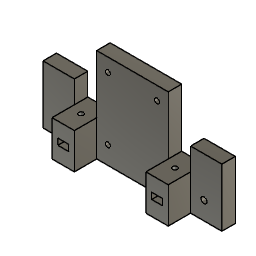
Y axis wheel frame v1 (Autodesk Fusion 360 design; units mm, degrees)
Autodesk Fusion 360 part; units mm, degrees
note: some values were not read from the file. Set by a fixed rule: which face or edge a step refers to.
sketch "Sketch1" plane through (0, 0, 0) normal (0, 1, 0) x (1, 0, 0)
  circle A0 centre (80, -25) radius 3.3
  circle A1 centre (-80, -25) radius 3.3
  line L0 (-100, -45) -> (-100, -5)
  line L1 (-100, -5) -> (100, -5)
  line L2 (100, -5) -> (100, -45)
  circle A2 centre (-80, -25) radius 6.55 construction
  circle A3 centre (80, -25) radius 6.55 construction
  line L3 (-65, -45) -> (-40, -45)
  line L4 (-40, -45) -> (-40, -5)
  line L5 (-40, -5) -> (-65, -5)
  line L6 (-65, -5) -> (-65, -45)
  line L7 (65, -45) -> (40, -45)
  line L8 (40, -45) -> (40, -5)
  line L9 (40, -5) -> (65, -5)
  line L10 (65, -5) -> (65, -45)
  line L11 (-40, -25) -> (-27.5, -25) construction
  line L12 (40, -25) -> (27.5, -25) construction
  circle A4 centre (-27.5, -25) radius 2.75
  circle A5 centre (27.5, -25) radius 2.75
  line L13 (-27.5, -25) -> (-27.5, -95) construction
  line L14 (27.5, -25) -> (27.5, -95) construction
  circle A6 centre (27.5, -95) radius 2.75
  circle A7 centre (-27.5, -95) radius 2.75
  line L15 (40, -45) -> (40, -105)
  line L16 (40, -105) -> (-40, -105)
  line L17 (-40, -105) -> (-40, -45)
  line L18 (-100, -45) -> (-65, -45)
  line L19 (65, -45) -> (100, -45)
  dimension "d3" = 160
  dimension "d4" = 6.6
  dimension "d5" = 6.6
  dimension "d6" = 13.1
  dimension "d7" = 13.1
  dimension "d11" = 12.5
  dimension "d12" = 12.5
  dimension "d13" = 5.5
  dimension "d14" = 5.5
  dimension "d15" = 70
  dimension "d16" = 70
  dimension "d17" = 5.5
  dimension "d18" = 5.5
  constraint vertical L0
  constraint horizontal L1
  constraint vertical L2
  constraint concentric A1 A2
  constraint concentric A0 A3
  constraint horizontal L3
  constraint vertical L4
  constraint horizontal L5
  constraint vertical L6
  constraint coincident L1 L4.end
  constraint horizontal L7
  constraint vertical L8
  constraint horizontal L9
  constraint vertical L10
  constraint coincident L1 L8.end
  constraint midpoint L4 L11.start
  constraint perpendicular L4 L11
  constraint midpoint L8 L12.start
  constraint perpendicular L8 L12
  constraint coincident L11.end A4.centre
  constraint coincident L12.end A5.centre
  constraint perpendicular L11 L13
  constraint coincident L14.end A6.centre
  constraint coincident L13.end A7.centre
  constraint vertical L15
  constraint horizontal L16
  constraint vertical L17
  constraint perpendicular L6 L18
  constraint perpendicular L2 L19
  measures "d3" distance of A0.centre A1.centre
  measures "d4" diameter of A0
  measures "d5" diameter of A1
  measures "d6" diameter of A2
  measures "d7" diameter of A3
  measures "d11" distance of L11.start L11.end
  measures "d12" distance of L12.start L12.end
  measures "d13" diameter of A4
  measures "d14" diameter of A5
  measures "d15" distance of L11.end L13.end
  measures "d16" distance of L12.end L14.end
  measures "d17" diameter of A6
  measures "d18" diameter of A7
extrude "Extrude1" add sketch "Sketch1" along normal blind 15
extrude "Extrude2" add sketch "Sketch1" against normal blind 85 contours L1 L3 L4 L5 L6 | L1 L7 L8 L9 L10
sketch "Sketch2" plane through (0, 0, 45) normal (0, 0, 1) x (-1, 0, 0)
  line L0 (100, 0) -> (65, 0)
  line L1 (65, 0) -> (65, 85)
  line L2 (65, 85) -> (40, 85)
  line L3 (40, 85) -> (40, 0)
  line L4 (40, 0) -> (40, -15)
  line L5 (40, -15) -> (100, -15)
  line L6 (100, -15) -> (100, 0)
  line L7 (65, 0) -> (40, 0) construction
  line L8 (52.5, -15) -> (52.5, 5) construction
  line L9 (52.5, 5) -> (52.5, 75) construction
  dimension "d23" = 20
  dimension "d24" = 70
  constraint coincident L0.end L1.start
  constraint coincident L3.end L4.start
  constraint coincident L5 L8.start
  constraint perpendicular L7 L8
  constraint parallel L8 L9
  measures "d23" distance of L8.start L8.end
  measures "d24" distance of L8.end L9.end
sketch "Sketch3" plane through (0, 0, 45) normal (0, 0, 1) x (-1, 0, 0)
  line L0 (-65, 0) -> (-100, 0)
  line L1 (-100, 0) -> (-100, -15)
  line L2 (-100, -15) -> (-40, -15)
  line L3 (-40, -15) -> (-40, 0)
  line L4 (-40, 0) -> (-40, 85)
  line L5 (-40, 85) -> (-65, 85)
  line L6 (-65, 85) -> (-65, 0)
  line L7 (-65, 0) -> (-40, 0) construction
  line L8 (-52.5, -15) -> (-52.5, 5) construction
  line L9 (-52.5, 5) -> (-52.5, 75) construction
  dimension "d25" = 20
  dimension "d26" = 70
  constraint coincident L0.start L6.end
  constraint coincident L3.end L4.start
  constraint coincident L2 L8.start
  constraint perpendicular L2 L8
  constraint perpendicular L2 L9
  measures "d25" distance of L8.start L8.end
  measures "d26" distance of L8.end L9.end
hole "Hole1" at (-52.5, -5, 45) at (52.5, -5, 45) direction (0, 0, -1) diameter 5.5 depth 40 tip angle 180
extrude "Extrude3" cut 2 faces at (-56.6667, -85, 18.3333) (48.3333, -85, 18.3333) along direction (0, 1, 0) blind 65
extrude "Extrude4" add 2 faces at (-56.6667, -20, 18.3333) (48.3333, -20, 18.3333) along direction (0, -1, 0) blind 5
extrude "Extrude5" add 1 faces at (13.3333, 5, 105) along direction (0, 0, 1) blind 5
sketch "Sketch4" plane through (0, 0, 45) normal (0, 0, 1) x (-1, 0, 0)
  line L0 (40, 25) -> (40, 0)
  line L1 (40, 0) -> (40, -15)
  line L2 (40, -15) -> (100, -15)
  line L3 (100, -15) -> (100, 0)
  line L4 (100, 0) -> (65, 0)
  line L5 (65, 0) -> (65, 25)
  line L6 (65, 25) -> (40, 25)
  circle A0 centre (52.5, 5) radius 2.75
  line L7 (65, 0) -> (65, -15)
  constraint coincident L4.end L5.start
  constraint coincident L2 L7.end
  constraint perpendicular L2 L7
sketch "Sketch5" plane through (0, 0, 45) normal (0, 0, 1) x (-1, 0, 0)
  line L0 (-65, 25) -> (-65, 0)
  line L1 (-65, 0) -> (-100, 0)
  line L2 (-100, 0) -> (-100, -15)
  line L3 (-100, -15) -> (-40, -15)
  line L4 (-40, -15) -> (-40, 0)
  line L5 (-40, 0) -> (-40, 25)
  line L6 (-40, 25) -> (-65, 25)
  circle A0 centre (-52.5, 5) radius 2.75
  line L7 (-65, 0) -> (-65, -15)
  constraint coincident L0.end L1.start
  constraint coincident L3 L7.end
  constraint perpendicular L3 L7
extrude "Extrude6" add sketch "Sketch5" sketch "Sketch4" along normal blind 25 contours L1 L2 L3 L7 of sketch 2 contours L2 L3 L4 L7
move_body "Move1" bodies 1 to x (1, 0, 0) y (0, 1, 0) z (0, 0, 1) at (0, 0, -5)
sketch "Sketch6" plane through (0, -25, 0) normal (0, -1, 0) x (1, 0, 0)
  line L0 (-65, 40) -> (-65, 0)
  line L1 (-65, 0) -> (-40, 0)
  line L2 (-40, 0) -> (-40, 40)
  line L3 (-40, 40) -> (-65, 40)
  line L4 (-65, 20) -> (-40, 20) construction
  line L5 (-52.5, 40) -> (-52.5, 0) construction
  line L6 (-46.5, 23.5) -> (-58.5, 23.5)
  line L7 (-58.5, 23.5) -> (-58.5, 16.5)
  line L8 (-58.5, 16.5) -> (-46.5, 16.5)
  line L9 (-46.5, 16.5) -> (-46.5, 23.5)
  dimension "d41" = 12
  dimension "d42" = 7
  constraint midpoint L0 L4.start
  constraint midpoint L2 L4.end
  constraint midpoint L3 L5.start
  constraint midpoint L1 L5.end
  constraint horizontal L6
  constraint vertical L7
  constraint horizontal L8
  constraint vertical L9
  measures "d41" distance of L6.start L6.end
  measures "d42" distance of L6.start L8.end
sketch "Sketch7" plane through (0, -25, 0) normal (0, -1, 0) x (1, 0, 0)
  line L0 (40, 0) -> (65, 0)
  line L1 (65, 0) -> (65, 40)
  line L2 (65, 40) -> (40, 40)
  line L3 (40, 40) -> (40, 0)
  line L4 (52.5, 40) -> (52.5, 0) construction
  line L5 (65, 20) -> (40, 20) construction
  line L6 (58.5, 23.5) -> (46.5, 23.5)
  line L7 (46.5, 23.5) -> (46.5, 16.5)
  line L8 (46.5, 16.5) -> (58.5, 16.5)
  line L9 (58.5, 16.5) -> (58.5, 23.5)
  dimension "d43" = 7
  dimension "d44" = 12
  constraint midpoint L2 L4.start
  constraint midpoint L0 L4.end
  constraint midpoint L1 L5.start
  constraint midpoint L3 L5.end
  constraint horizontal L6
  constraint vertical L7
  constraint horizontal L8
  constraint vertical L9
  measures "d43" distance of L6.start L8.end
  measures "d44" distance of L6.start L6.end
delete_face "DeleteFace1" 2 faces at (-52.3629, -7.7466, 26.6667) (52.6371, -7.7466, 26.6667)
extrude "Extrude7" cut sketch "Sketch6" sketch "Sketch7" against normal blind 20 contours L6 L7 L8 L9 of sketch 2 contours L6 L7 L8 L9
extrude "Extrude8" cut 2 faces at (-54.5, -5, 21.1667) (50.5, -5, 21.1667) along direction (0, 1, 0) blind 6
chamfer "Chamfer1" distance 3 angle 45 4 edges at (58.5, 1, 20) (46.5, 1, 20) (-58.5, 1, 20) (-46.5, 1, 20)
extrude "Extrude10" cut sketch "Sketch5" sketch "Sketch4" against normal blind 21.5 contours A0 of sketch 2 contours A0
